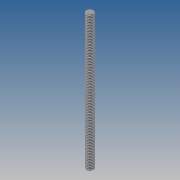
# Autodesk Inventor part: M8 LEAD SCREW
Saved by Autodesk Inventor 2013 (Build 170138000, 138)
## iProperties
Created: 2017-04-04
Part Number: M8 LEAD SCREW
Material: Generic
Document SubType Name: Modeling
Designer: employee
Density: 1 g/cm^3
Author: employee
Autodesk Inventor part; units mm, degrees
ref_plane "YZ Plane" through (0, 0, 0) normal (1, 0, 0) x (0, 1, 0)
ref_plane "XZ Plane" through (0, 0, 0) normal (0, 1, 0) x (-1, 0, 0)
ref_plane "XY Plane" through (0, 0, 0) normal (0, 0, 1) x (1, 0, 0)
sketch "Sketch1" plane through (0, 0, 0) normal (0, 0, 1) x (1, 0, 0)
  circle A0 centre (0, 0) radius 4
  dimension "d0" = 8
  constraints: 1 centre point, 1 coincident
  measures "d0" diameter of A0
extrude "Extrusion1" add sketch "Sketch1" along normal blind 150
sketch "Sketch2" plane through (0, 0, 0) normal (1, 0, 0) x (0, 1, 0)
  line L0 (4, 150) -> (4, 0) projected
  line L1 (4, 0) -> (-4, 0) projected
  line L2 (-4, 0) -> (-4, 150) projected
  line L3 (-4, 150) -> (4, 150) projected
  line L4 (-4, 0) -> (-4, -0.9569)
  line L5 (-4, -0.9569) -> (-3.2, -0.75)
  line L6 (-3.2, -0.75) -> (-3.2, -0.2069)
  line L7 (-3.2, -0.2069) -> (-4, 0)
  line L8 (-3.6, -0.8534) -> (-3.6, -0.1034) construction
  point P0 (0, 0)
  dimension "d4" = 29
  dimension "d5" = 0.8
  dimension "d7" = 0.75
  constraints: 10 end point, 2 midpoint, 1 equal length, 1 parallel, 1 perpendicular
  measures "d4" angle of L7 L5
  measures "d5" distance between parallel lines of L6 L4
  measures "d7" distance of L8.start L8.end
coil "Coil1" sketch "Sketch2" operation cut axis through (0, 0, -10) along (0, 0, 1) pitch 1.5 turns 133.333333 hand right contours L7 L6 L5 L4
body "Solid1"
